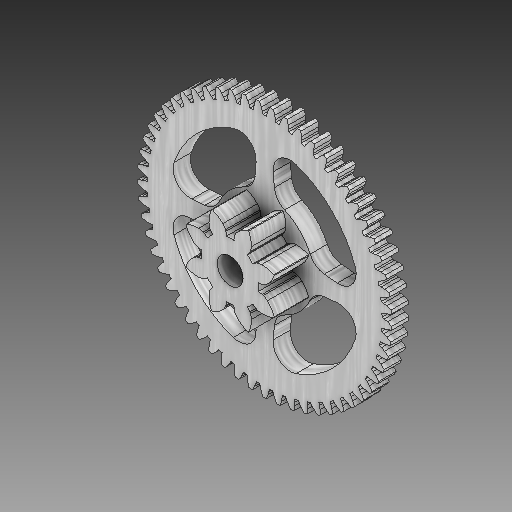
# Autodesk Inventor part: 多段ギアm1.z57,m2.z8
Saved by Autodesk Inventor 2020 (Build 240168000, 168)
## iProperties
Created: 2019-09-05
Part Number: 多段ギアm1.z57,m2.z8
Material: アルミニウム 7075
Document SubType Name: Modeling
Designer: 雪村
Density: 2.81 g/cm^3
Appearance: サテン - ブラシ仕上げ 重厚
Mass: 22.8746 g
Surface Area: 66.3884 cm^2
Volume: 8.14042 cm^3
Description: アルミ7000 12t
Author: 雪村
Autodesk Inventor part; units mm, degrees
(part 1 of 2)
ref_plane "YZ Plane" through (0, 0, 0) normal (1, 0, 0) x (0, 1, 0)
ref_plane "XZ Plane" through (0, 0, 0) normal (0, 1, 0) x (-1, 0, 0)
ref_plane "XY Plane" through (0, 0, 0) normal (0, 0, 1) x (1, 0, 0)
sketch "スケッチ1" plane through (0, 0, 0) normal (0, 0, 1) x (1, 0, 0)
  arc A0 (1.0775, 7.7333) -> (0.985, 7.4527) centre (2.1428, 7.2265) ccw
  arc A1 (1.6924, 8.6387) -> (1.0775, 7.7333) centre (4.1275, 6.3233) ccw
  arc A2 (4.1322, 10.2254) -> (1.6924, 8.6387) centre (6.2553, 4.2918) ccw
  arc A3 (-4.7064, 6.2301) -> (-4.5734, 5.9664) centre (-3.5947, 6.6251) ccw
  arc A4 (-4.9118, 7.3052) -> (-4.7064, 6.2301) centre (-1.5527, 7.3898) ccw
  arc A5 (-4.3085, 10.1524) -> (-4.9118, 7.3052) centre (1.3884, 7.4579) ccw
  arc A6 (-7.7333, 1.0775) -> (-7.4527, 0.985) centre (-7.2265, 2.1428) ccw
  arc A7 (-8.6387, 1.6924) -> (-7.7333, 1.0775) centre (-6.3233, 4.1275) ccw
  arc A8 (-10.2254, 4.1322) -> (-8.6387, 1.6924) centre (-4.2918, 6.2553) ccw
  arc A9 (-6.2301, -4.7064) -> (-5.9664, -4.5734) centre (-6.6251, -3.5947) ccw
  arc A10 (-7.3052, -4.9118) -> (-6.2301, -4.7064) centre (-7.3898, -1.5527) ccw
  arc A11 (-10.1524, -4.3085) -> (-7.3052, -4.9118) centre (-7.4579, 1.3884) ccw
  arc A12 (-1.0775, -7.7333) -> (-0.985, -7.4527) centre (-2.1428, -7.2265) ccw
  arc A13 (-1.6924, -8.6387) -> (-1.0775, -7.7333) centre (-4.1275, -6.3233) ccw
  arc A14 (-4.1322, -10.2254) -> (-1.6924, -8.6387) centre (-6.2553, -4.2918) ccw
  arc A15 (4.7064, -6.2301) -> (4.5734, -5.9664) centre (3.5947, -6.6251) ccw
  arc A16 (4.9118, -7.3052) -> (4.7064, -6.2301) centre (1.5527, -7.3898) ccw
  arc A17 (4.3085, -10.1524) -> (4.9118, -7.3052) centre (-1.3884, -7.4579) ccw
  arc A18 (7.7333, -1.0775) -> (7.4527, -0.985) centre (7.2265, -2.1428) ccw
  arc A19 (8.6387, -1.6924) -> (7.7333, -1.0775) centre (6.3233, -4.1275) ccw
  arc A20 (10.2254, -4.1322) -> (8.6387, -1.6924) centre (4.2918, -6.2553) ccw
  arc A21 (6.2301, 4.7064) -> (5.9664, 4.5734) centre (6.6251, 3.5947) ccw
  arc A22 (7.3052, 4.9118) -> (6.2301, 4.7064) centre (7.3898, 1.5527) ccw
  arc A23 (10.1524, 4.3085) -> (7.3052, 4.9118) centre (7.4579, -1.3884) ccw
  arc A24 (-0.985, 7.4527) -> (-1.0775, 7.7333) centre (-2.1428, 7.2265) ccw
  arc A25 (-1.0775, 7.7333) -> (-1.6924, 8.6387) centre (-4.1275, 6.3233) ccw
  arc A26 (-1.6924, 8.6387) -> (-4.1322, 10.2254) centre (-6.2553, 4.2918) ccw
  arc A27 (-5.9664, 4.5734) -> (-6.2301, 4.7064) centre (-6.6251, 3.5947) ccw
  arc A28 (-6.2301, 4.7064) -> (-7.3052, 4.9118) centre (-7.3898, 1.5527) ccw
  arc A29 (-7.3052, 4.9118) -> (-10.1524, 4.3085) centre (-7.4579, -1.3884) ccw
  arc A30 (-7.4527, -0.985) -> (-7.7333, -1.0775) centre (-7.2265, -2.1428) ccw
  arc A31 (-7.7333, -1.0775) -> (-8.6387, -1.6924) centre (-6.3233, -4.1275) ccw
  arc A32 (-8.6387, -1.6924) -> (-10.2254, -4.1322) centre (-4.2918, -6.2553) ccw
  arc A33 (-4.5734, -5.9664) -> (-4.7064, -6.2301) centre (-3.5947, -6.6251) ccw
  arc A34 (-4.7064, -6.2301) -> (-4.9118, -7.3052) centre (-1.5527, -7.3898) ccw
  arc A35 (-4.9118, -7.3052) -> (-4.3085, -10.1524) centre (1.3884, -7.4579) ccw
  arc A36 (0.985, -7.4527) -> (1.0775, -7.7333) centre (2.1428, -7.2265) ccw
  arc A37 (1.0775, -7.7333) -> (1.6924, -8.6387) centre (4.1275, -6.3233) ccw
  arc A38 (1.6924, -8.6387) -> (4.1322, -10.2254) centre (6.2553, -4.2918) ccw
  arc A39 (5.9664, -4.5734) -> (6.2301, -4.7064) centre (6.6251, -3.5947) ccw
  arc A40 (6.2301, -4.7064) -> (7.3052, -4.9118) centre (7.3898, -1.5527) ccw
  arc A41 (7.3052, -4.9118) -> (10.1524, -4.3085) centre (7.4579, 1.3884) ccw
  arc A42 (7.4527, 0.985) -> (7.7333, 1.0775) centre (7.2265, 2.1428) ccw
  arc A43 (7.7333, 1.0775) -> (8.6387, 1.6924) centre (6.3233, 4.1275) ccw
  arc A44 (8.6387, 1.6924) -> (10.2254, 4.1322) centre (4.2918, 6.2553) ccw
  arc A45 (4.5734, 5.9664) -> (4.7064, 6.2301) centre (3.5947, 6.6251) ccw
  arc A46 (4.7064, 6.2301) -> (4.9118, 7.3052) centre (1.5527, 7.3898) ccw
  arc A47 (4.9118, 7.3052) -> (4.3085, 10.1524) centre (-1.3884, 7.4579) ccw
  arc A48 (0.8647, 6.5431) -> (-0.8647, 6.5431) centre (0, 0) ccw
  arc A49 (-4.0152, 5.2381) -> (-5.2381, 4.0152) centre (0, 0) ccw
  arc A50 (-6.5431, 0.8647) -> (-6.5431, -0.8647) centre (0, 0) ccw
  arc A51 (-5.2381, -4.0152) -> (-4.0152, -5.2381) centre (0, 0) ccw
  arc A52 (-0.8647, -6.5431) -> (0.8647, -6.5431) centre (0, 0) ccw
  arc A53 (4.0152, -5.2381) -> (5.2381, -4.0152) centre (0, 0) ccw
  arc A54 (6.5431, -0.8647) -> (6.5431, 0.8647) centre (0, 0) ccw
  arc A55 (5.2381, 4.0152) -> (4.0152, 5.2381) centre (0, 0) ccw
  arc A56 (-4.1322, 10.2254) -> (-4.3085, 10.1524) centre (0, 0) ccw
  arc A57 (-10.1524, 4.3085) -> (-10.2254, 4.1322) centre (0, 0) ccw
  arc A58 (-10.2254, -4.1322) -> (-10.1524, -4.3085) centre (0, 0) ccw
  arc A59 (-4.3085, -10.1524) -> (-4.1322, -10.2254) centre (0, 0) ccw
  arc A60 (4.1322, -10.2254) -> (4.3085, -10.1524) centre (0, 0) ccw
  arc A61 (10.1524, -4.3085) -> (10.2254, -4.1322) centre (0, 0) ccw
  arc A62 (10.2254, 4.1322) -> (10.1524, 4.3085) centre (0, 0) ccw
  arc A63 (4.3085, 10.1524) -> (4.1322, 10.2254) centre (0, 0) ccw
  line L0 (0.8647, 6.5431) -> (0.985, 7.4527)
  line L1 (-4.0152, 5.2381) -> (-4.5734, 5.9664)
  line L2 (-6.5431, 0.8647) -> (-7.4527, 0.985)
  line L3 (-5.2381, -4.0152) -> (-5.9664, -4.5734)
  line L4 (-0.8647, -6.5431) -> (-0.985, -7.4527)
  line L5 (4.0152, -5.2381) -> (4.5734, -5.9664)
  line L6 (6.5431, -0.8647) -> (7.4527, -0.985)
  line L7 (5.2381, 4.0152) -> (5.9664, 4.5734)
  line L8 (-0.8647, 6.5431) -> (-0.985, 7.4527)
  line L9 (-5.2381, 4.0152) -> (-5.9664, 4.5734)
  line L10 (-6.5431, -0.8647) -> (-7.4527, -0.985)
  line L11 (-4.0152, -5.2381) -> (-4.5734, -5.9664)
  line L12 (0.8647, -6.5431) -> (0.985, -7.4527)
  line L13 (5.2381, -4.0152) -> (5.9664, -4.5734)
  line L14 (6.5431, 0.8647) -> (7.4527, 0.985)
  line L15 (4.0152, 5.2381) -> (4.5734, 5.9664)
  line L16 (-13.0288, 0) -> (13.0288, 0)
  line L17 (0, -13.0288) -> (0, 13.0288)
  line L18 (31.0288, 11.0288) -> (101.0288, 11.0288)
  line L19 (31.0288, 3.0288) -> (101.0288, 3.0288)
  line L20 (31.0288, -4.9712) -> (101.0288, -4.9712)
  line L21 (31.0288, -12.9712) -> (101.0288, -12.9712)
  line L22 (31.0288, -20.9712) -> (101.0288, -20.9712)
  line L23 (31.0288, -28.9712) -> (101.0288, -28.9712)
  line L24 (31.0288, -36.9712) -> (101.0288, -36.9712)
  line L25 (31.0288, -44.9712) -> (101.0288, -44.9712)
  line L26 (31.0288, -52.9712) -> (101.0288, -52.9712)
  line L27 (31.0288, -60.9712) -> (101.0288, -60.9712)
  line L28 (31.0288, -68.9712) -> (101.0288, -68.9712)
  line L29 (31.0288, -76.9712) -> (101.0288, -76.9712)
  line L30 (31.0288, -84.9712) -> (101.0288, -84.9712)
  line L31 (31.0288, 11.0288) -> (31.0288, -84.9712)
  line L32 (101.0288, 11.0288) -> (101.0288, -84.9712)
  line L33 (66.0288, 3.0288) -> (66.0288, -84.9712)
  point P0 (0, 0)
  point P1 (37.0288, 5.0288)
  point P2 (39.5288, -2.9712)
  point P3 (39.5288, -10.9712)
  point P4 (37.0288, -18.9712)
  point P5 (39.5288, -26.9712)
  point P6 (34.5288, -34.9712)
  point P7 (37.0288, -42.9712)
  point P8 (37.0288, -50.9712)
  point P9 (37.0288, -58.9712)
  point P10 (39.5288, -66.9712)
  point P11 (39.5288, -74.9712)
  point P12 (37.0288, -82.9712)
  point P13 (67.0288, -2.9712)
  point P14 (83.2788, -10.9712)
  point P15 (83.2788, -18.9712)
  point P16 (79.5288, -26.9712)
  point P17 (82.0288, -34.9712)
  point P18 (75.7788, -42.9712)
  point P19 (75.7788, -50.9712)
  point P20 (79.5288, -58.9712)
  point P21 (77.0288, -66.9712)
  point P22 (1, 26.5288)
  point P23 (1, 20.5288)
  point P24 (18.25, 26.5288)
  point P25 (20.375, 20.5288)
  constraints: 128 point on circle, 64 centre point, 64 end point, 14 horizontal, 2 midpoint, 2 vertical, 320 other
extrude "押し出し1" add sketch "スケッチ1" along normal blind 8 contours A1 A2 A63 A47 A46 A45 L15 A55 L7 A21 A22 A23 A62 A44 A43 A42 L14 A54 L16 L17 A48 L0 A0 | L17 L16 A50 L2 A6 A7 A8 A57 A29 A28 A27 L9 A49 L1 A3 A4 A5 A56 A26 A25 A24 L8 A48 | L17 A52 L4 A12 A13 A14 A59 A35 A34 A33 L11 A51 L3 A9 A10 A11 A58 A32 A31 A30 L10 A50 L16 | L16 A54 L6 A18 A19 A20 A61 A41 A40 A39 L13 A53 L5 A15 A16 A17 A60 A38 A37 A36 L12 A52 L17
sketch "スケッチ2" plane through (0, 0, 0) normal (0, 0, -1) x (-1, 0, 0)
  arc A0 (0.535, 27.768) -> (0.4038, 27.247) centre (6.485, 25.9929) ccw
  arc A1 (0.7907, 28.5027) -> (0.535, 27.768) centre (8.7588, 25.3182) ccw
  arc A2 (1.2341, 29.4742) -> (0.7907, 28.5027) centre (11.0839, 24.3913) ccw
  arc A3 (-2.523, 27.6583) -> (-2.596, 27.1261) centre (3.5862, 26.5485) ccw
  arc A4 (-2.3497, 28.4167) -> (-2.523, 27.6583) centre (5.9205, 26.128) ccw
  arc A5 (-2.0158, 29.431) -> (-2.3497, 28.4167) centre (8.3334, 25.4626) ccw
  arc A6 (-5.5503, 27.2129) -> (-5.5644, 26.6758) centre (0.6439, 26.7819) ccw
  arc A7 (-5.4615, 27.9857) -> (-5.5503, 27.2129) centre (3.0102, 26.6208) ccw
  arc A8 (-5.2412, 29.0307) -> (-5.4615, 27.9857) centre (5.4817, 26.2248) ccw
  arc A9 (-8.5102, 26.4372) -> (-8.4651, 25.9018) centre (-2.3063, 26.6901) ccw
  arc A10 (-8.507, 27.2151) -> (-8.5102, 26.4372) centre (0.0635, 26.7903) ccw
  arc A11 (-8.403, 28.2779) -> (-8.507, 27.2151) centre (2.5635, 26.6687) ccw
  arc A12 (-11.3669, 25.3405) -> (-11.2632, 24.8134) centre (-5.2284, 26.2744) ccw
  arc A13 (-11.4492, 26.1141) -> (-11.3669, 25.3405) centre (-2.8841, 26.6347) ccw
  arc A14 (-11.4628, 27.1819) -> (-11.4492, 26.1141) centre (-0.3858, 26.7888) ccw
  arc A15 (-14.0856, 23.9363) -> (-13.9245, 23.4237) centre (-8.0871, 25.5398) ccw
  arc A16 (-14.2525, 24.6961) -> (-14.0856, 23.9363) centre (-5.7966, 26.1558) ccw
  arc A17 (-14.3835, 25.7559) -> (-14.2525, 24.6961) centre (-3.3305, 26.5838) ccw
  arc A18 (-16.6333, 22.2415) -> (-16.4168, 21.7498) centre (-10.8476, 24.4952) ccw
  arc A19 (-16.8828, 22.9783) -> (-16.6333, 22.2415) centre (-8.6388, 25.3594) ccw
  arc A20 (-17.1295, 24.0173) -> (-16.8828, 22.9783) centre (-6.2347, 26.0561) ccw
  arc A21 (-18.9791, 20.2767) -> (-18.7098, 19.8118) centre (-13.4764, 23.1532) ccw
  arc A22 (-19.3081, 20.9816) -> (-18.9791, 20.2767) centre (-11.3761, 24.2551) ccw
  arc A23 (-19.6677, 21.9871) -> (-19.3081, 20.9816) centre (-9.0632, 25.2121) ccw
  arc A24 (-21.0945, 18.0658) -> (-20.7757, 17.6333) centre (-15.9417, 21.5301) ccw
  arc A25 (-21.4991, 18.7302) -> (-21.0945, 18.0658) centre (-13.9753, 22.8564) ccw
  arc A26 (-21.9671, 19.69) -> (-21.4991, 18.7302) centre (-11.7818, 24.062) ccw
  arc A27 (-22.9538, 15.6355) -> (-22.5894, 15.2408) centre (-18.2134, 19.6457) ccw
  arc A28 (-23.4291, 16.2514) -> (-22.9538, 15.6355) centre (-16.4049, 21.1803) ccw
  arc A29 (-23.9998, 17.154) -> (-23.4291, 16.2514) centre (-14.3573, 22.6199) ccw
  arc A30 (-24.5345, 13.0155) -> (-24.1289, 12.6632) centre (-20.2641, 17.5229) ccw
  arc A31 (-25.0747, 13.5754) -> (-24.5345, 13.0155) centre (-18.6353, 19.2471) ccw
  arc A32 (-25.7412, 14.4097) -> (-25.0747, 13.5754) centre (-16.7585, 20.9032) ccw
  arc A33 (-25.8175, 10.2375) -> (-25.3755, 9.932) centre (-22.0687, 15.1873) ccw
  arc A34 (-26.4159, 10.7346) -> (-25.8175, 10.2375) centre (-20.6396, 17.0802) ccw
  arc A35 (-27.1702, 11.4905) -> (-26.4159, 10.7346) centre (-18.9563, 18.9327) ccw
  arc A36 (-26.787, 7.3353) -> (-26.3141, 7.0802) centre (-23.6055, 12.6674) ccw
  arc A37 (-27.4364, 7.7635) -> (-26.787, 7.3353) centre (-22.3933, 14.7061) ccw
  arc A38 (-28.2693, 8.4318) -> (-27.4364, 7.7635) centre (-20.924, 16.7325) ccw
  arc A39 (-27.4313, 4.344) -> (-26.9333, 4.1425) centre (-24.8558, 9.9937) ccw
  arc A40 (-28.124, 4.6981) -> (-27.4313, 4.344) centre (-23.8751, 12.1534) ccw
  arc A41 (-29.0253, 5.2708) -> (-28.124, 4.6981) centre (-22.6377, 14.3291) ccw
  arc A42 (-27.7427, 1.2999) -> (-27.2255, 1.1544) centre (-25.8043, 7.1987) ccw
  arc A43 (-28.4701, 1.5757) -> (-27.7427, 1.2999) centre (-25.0672, 9.4531) ccw
  arc A44 (-29.429, 2.0458) -> (-28.4701, 1.5757) centre (-24.0767, 11.7518) ccw
  arc A45 (-27.7173, -1.7599) -> (-27.1873, -1.8476) centre (-26.4396, 4.3163) ccw
  arc A46 (-28.4707, -1.5658) -> (-27.7173, -1.7599) centre (-25.955, 6.6382) ccw
  arc A47 (-29.4754, -1.2041) -> (-28.4707, -1.5658) centre (-25.2233, 9.0318) ccw
  arc A48 (-27.3555, -4.7983) -> (-26.819, -4.8272) centre (-26.754, 1.3816) ccw
  arc A49 (-28.1256, -4.6883) -> (-27.3555, -4.7983) centre (-26.5277, 3.7426) ccw
  arc A50 (-29.1641, -4.4393) -> (-28.1256, -4.6883) centre (-26.0638, 6.2023) ccw
  arc A51 (-26.6616, -7.7786) -> (-26.1252, -7.7482) centre (-26.7436, -1.57) ccw
  arc A52 (-27.4392, -7.7539) -> (-26.6616, -7.7786) centre (-26.7784, 0.8016) ccw
  arc A53 (-28.4987, -7.6207) -> (-27.4392, -7.7539) centre (-26.5879, 3.2974) ccw
  arc A54 (-25.6441, -10.6643) -> (-25.1143, -10.5752) centre (-26.4085, -4.5025) ccw
  arc A55 (-26.4196, -10.7253) -> (-25.6441, -10.6643) centre (-26.7041, -2.1491) ccw
  arc A56 (-27.4874, -10.7095) -> (-26.4196, -10.7253) centre (-26.7893, 0.3525) ccw
  arc A57 (-24.3153, -13.4207) -> (-23.7985, -13.2738) centre (-25.7529, -7.3803) ccw
  arc A58 (-25.0794, -13.5666) -> (-24.3153, -13.4207) centre (-26.3056, -5.0737) ccw
  arc A59 (-26.1424, -13.6683) -> (-25.0794, -13.5666) centre (-26.6655, -2.5967) ccw
  arc A60 (-22.6913, -16.0141) -> (-22.1938, -15.8113) centre (-24.7848, -10.1685) ccw
  arc A61 (-23.4347, -16.2432) -> (-22.6913, -16.0141) centre (-25.5878, -7.9368) ccw
  arc A62 (-24.4801, -16.4613) -> (-23.4347, -16.2432) centre (-26.218, -5.5144) ccw
  arc A63 (-20.7919, -18.4131) -> (-20.3198, -18.1568) centre (-23.5157, -12.8333) ccw
  arc A64 (-21.5056, -18.7227) -> (-20.7919, -18.4131) centre (-24.5594, -10.7034) ccw
  arc A65 (-22.5207, -19.0544) -> (-21.5056, -18.7227) centre (-25.4522, -8.3651) ccw
  arc A66 (-18.6401, -20.5887) -> (-18.1991, -20.2819) centre (-21.9612, -15.3424) ccw
  arc A67 (-19.3155, -20.9748) -> (-18.6401, -20.5887) centre (-23.2328, -13.3402) ccw
  arc A68 (-20.2879, -21.4162) -> (-19.3155, -20.9748) centre (-24.3775, -11.1143) ccw
  arc A69 (-16.2621, -22.5143) -> (-15.8574, -22.1609) centre (-20.1401, -17.6652) ccw
  arc A70 (-16.8908, -22.9724) -> (-16.2621, -22.5143) centre (-21.6243, -15.8151) ccw
  arc A71 (-17.8088, -23.518) -> (-16.8908, -22.9724) centre (-23.0069, -13.7285) ccw
  arc A72 (-13.6866, -24.1666) -> (-13.3233, -23.7708) centre (-18.0746, -19.7735) ccw
  arc A73 (-14.2612, -24.6911) -> (-13.6866, -24.1666) centre (-19.7533, -18.0979) ccw
  arc A74 (-15.1135, -25.3344) -> (-14.2612, -24.6911) centre (-21.357, -16.1762) ccw
  arc A75 (-10.945, -25.5256) -> (-10.6274, -25.0922) centre (-15.7896, -21.6419) ccw
  arc A76 (-11.4584, -26.1101) -> (-10.945, -25.5256) centre (-17.6425, -20.1611) ccw
  arc A77 (-12.2348, -26.8433) -> (-11.4584, -26.1101) centre (-19.4479, -18.4274) ccw
  arc A78 (-8.0706, -26.5747) -> (-7.8026, -26.109) centre (-13.313, -23.2475) ccw
  arc A79 (-8.5165, -27.2121) -> (-8.0706, -26.5747) centre (-15.3175, -21.9796) ccw
  arc A80 (-9.2075, -28.0263) -> (-8.5165, -27.2121) centre (-17.3027, -20.455) ccw
  arc A81 (-5.0982, -27.3012) -> (-4.883, -26.8089) centre (-10.6748, -24.571) ccw
  arc A82 (-5.4713, -27.9838) -> (-5.0982, -27.3012) centre (-12.8066, -23.5312) ccw
  arc A83 (-6.0685, -28.8691) -> (-5.4713, -27.9838) centre (-14.9474, -22.2343) ccw
  arc A84 (-2.0639, -27.6964) -> (-1.9042, -27.1834) centre (-7.907, -25.5961) ccw
  arc A85 (-2.3596, -28.4159) -> (-2.0639, -27.6964) centre (-10.1402, -24.7972) ccw
  arc A86 (-2.8559, -29.3614) -> (-2.3596, -28.4159) centre (-12.4108, -23.7437) ccw
  arc A87 (0.9955, -27.7553) -> (1.0978, -27.2279) centre (-5.0432, -26.3106) ccw
  arc A88 (0.7807, -28.503) -> (0.9955, -27.7553) centre (-7.3508, -25.7622) ccw
  arc A89 (0.3915, -29.4974) -> (0.7807, -28.503) centre (-9.7234, -24.9649) ccw
  arc A90 (4.0428, -27.4773) -> (4.0864, -26.9419) centre (-2.1182, -26.7057) ccw
  arc A91 (3.9115, -28.2441) -> (4.0428, -27.4773) centre (-4.4721, -26.4145) ccw
  arc A92 (3.634, -29.2753) -> (3.9115, -28.2441) centre (-6.9181, -25.883) ccw
  arc A93 (7.041, -26.8658) -> (7.0254, -26.3288) centre (0.8325, -26.7767) ccw
  arc A94 (6.9957, -27.6348) -> (7.041, -26.8658) centre (-1.5392, -26.7462) ccw
  arc A95 (6.8325, -28.6979) -> (6.9957, -27.6348) centre (-4.0287, -26.487) ccw
  arc A96 (9.9537, -25.9282) -> (9.8792, -25.3962) centre (3.7731, -26.5226) ccw
  arc A97 (9.9933, -26.7051) -> (9.9537, -25.9282) centre (1.4125, -26.7532) ccw
  arc A98 (9.948, -27.772) -> (9.9933, -26.7051) centre (-1.0905, -26.7694) ccw
  arc A99 (12.7456, -24.6759) -> (12.613, -24.1552) centre (6.6679, -25.9465) ccw
  arc A100 (12.8704, -25.4437) -> (12.7456, -24.6759) centre (4.347, -26.4354) ccw
  arc A101 (12.9428, -26.5091) -> (12.8704, -25.4437) centre (1.861, -26.7269) ccw
  arc A102 (15.3828, -23.124) -> (15.1937, -22.6211) centre (9.4817, -25.0555) ccw
  arc A103 (15.5913, -23.8734) -> (15.3828, -23.124) centre (7.2287, -25.7968) ccw
  arc A104 (15.7805, -24.9244) -> (15.5913, -23.8734) centre (4.7899, -26.36) ccw
  arc A105 (17.8332, -21.2914) -> (17.59, -20.8124) centre (12.1805, -23.8604) ccw
  arc A106 (18.123, -22.0133) -> (17.8332, -21.2914) centre (10.0227, -24.845) ccw
  arc A107 (18.4266, -23.0372) -> (18.123, -22.0133) centre (7.6606, -25.6731) ccw
  arc A108 (20.0672, -19.2004) -> (19.7728, -18.751) centre (14.7314, -22.3756) ccw
  arc A109 (20.4346, -19.8861) -> (20.0672, -19.2004) centre (12.695, -23.5916) ccw
  arc A110 (20.849, -20.8703) -> (20.4346, -19.8861) centre (10.4383, -24.6745) ccw
  arc A111 (22.0576, -16.8763) -> (21.7155, -16.462) centre (17.1035, -20.6192) ccw
  arc A112 (22.4982, -17.5174) -> (22.0576, -16.8763) centre (15.2132, -22.0519) ccw
  arc A113 (23.0184, -18.45) -> (22.4982, -17.5174) centre (13.0894, -23.3764) ccw
  arc A114 (23.7803, -14.3473) -> (23.3947, -13.9732) centre (19.268, -18.6126) ccw
  arc A115 (24.2887, -14.9361) -> (23.7803, -14.3473) centre (17.5468, -20.2445) ccw
  arc A116 (24.9083, -15.8058) -> (24.2887, -14.9361) centre (15.5815, -21.7946) ccw
  arc A117 (25.2143, -11.6442) -> (24.7899, -11.3148) centre (21.1986, -16.38) ccw
  arc A118 (25.7844, -12.1735) -> (25.2143, -11.6442) centre (19.6673, -18.1913) ccw
  arc A119 (26.4959, -12.9698) -> (25.7844, -12.1735) centre (17.8846, -19.9482) ccw
  arc A120 (26.3422, -8.7998) -> (25.8841, -8.519) centre (22.8719, -13.9485) ccw
  arc A121 (26.9671, -9.2631) -> (26.3422, -8.7998) centre (21.5491, -15.9173) ccw
  arc A122 (27.7619, -9.9763) -> (26.9671, -9.2631) centre (19.9705, -17.8597) ccw
  arc A123 (27.1504, -5.8485) -> (26.6642, -5.6199) centre (24.2675, -11.3478) ccw
  arc A124 (27.8224, -6.2403) -> (27.1504, -5.8485) centre (23.1694, -13.4501) ccw
  arc A125 (28.6909, -6.8617) -> (27.8224, -6.2403) centre (21.814, -15.5544) ccw
  arc A126 (27.629, -2.8262) -> (27.1206, -2.6525) centre (25.3685, -8.6093) ccw
  arc A127 (28.3401, -3.1417) -> (27.629, -2.8262) centre (24.5084, -10.8197) ccw
  arc A128 (29.2716, -3.6638) -> (28.3401, -3.1417) centre (23.3927, -13.0603) ccw
  arc A129 (27.7722, 0.2303) -> (27.2478, 0.3471) centre (26.1617, -5.7663) ccw
  arc A130 (28.5137, -0.005) -> (27.7722, 0.2303) centre (25.5499, -8.0579) ccw
  arc A131 (29.497, -0.4215) -> (28.5137, -0.005) centre (24.6875, -10.4076) ccw
  arc A132 (27.5783, 3.2841) -> (27.0442, 3.3425) centre (26.6372, -2.8533) ccw
  arc A133 (28.3412, 3.1318) -> (27.5783, 3.2841) centre (26.2813, -5.1983) ccw
  arc A134 (29.3643, 2.826) -> (28.3412, 3.1318) centre (25.6826, -7.6286) ccw
  arc A135 (27.0496, 6.298) -> (26.5124, 6.2973) centre (26.7894, 0.0943) ccw
  arc A136 (27.8246, 6.2305) -> (27.0496, 6.298) centre (26.6936, -2.2756) ccw
  arc A137 (28.8752, 6.0392) -> (27.8246, 6.2305) centre (26.3659, -4.757) ccw
  arc A138 (26.1926, 9.2355) -> (25.6587, 9.1756) centre (26.6165, 3.0408) ccw
  arc A139 (26.9703, 9.2537) -> (26.1926, 9.2355) centre (26.7819, 0.6748) ccw
  arc A140 (28.0356, 9.179) -> (26.9703, 9.2537) centre (26.7292, -1.8277) ccw
  arc A141 (25.0177, 12.0608) -> (24.4936, 11.9426) centre (26.1204, 5.9504) ccw
  arc A142 (25.7887, 12.1645) -> (25.0177, 12.0608) centre (26.5451, 3.6169) ccw
  arc A143 (26.8557, 12.2075) -> (25.7887, 12.1645) centre (26.768, 1.1238) ccw
  arc A144 (23.5391, 14.7398) -> (23.0312, 14.5646) centre (25.3073, 8.7878) ccw
  arc A145 (24.294, 14.9276) -> (23.5391, 14.7398) centre (25.9861, 6.5151) ccw
  arc A146 (25.3498, 15.0877) -> (24.294, 14.9276) centre (26.4819, 4.0617) ccw
  arc A147 (21.7747, 17.2398) -> (21.2891, 17.0099) centre (24.187, 11.5184) ccw
  arc A148 (22.4971, 17.5072) -> (21.7747, 17.2398) centre (25.1117, 9.3343) ccw
  arc A149 (23.5361, 17.7848) -> (22.4971, 17.5072) centre (25.8744, 6.9503) ccw
  arc A150 (19.746, 19.5306) -> (19.2887, 19.2486) centre (22.773, 14.1093) ccw
  arc A151 (20.4346, 19.8758) -> (19.746, 19.5306) centre (23.9325, 12.0401) ccw
  arc A152 (21.4368, 20.2661) -> (20.4346, 19.8758) centre (24.9528, 9.7545) ccw
  arc A153 (17.4777, 21.5843) -> (17.0541, 21.2537) centre (21.0827, 16.5289) ccw
  arc A154 (18.1241, 22.0031) -> (17.4777, 21.5843) centre (22.4627, 14.5998) ccw
  arc A155 (19.0773, 22.5013) -> (18.1241, 22.0031) centre (23.7282, 12.4403) ccw
  arc A156 (14.9971, 23.3759) -> (14.6125, 23.0008) centre (19.1364, 18.7478) ccw
  arc A157 (15.5935, 23.8634) -> (14.9971, 23.3759) centre (20.7203, 16.9823) ccw
  arc A158 (16.4862, 24.4634) -> (15.5935, 23.8634) centre (22.2157, 14.9751) ccw
  arc A159 (12.3346, 24.8839) -> (11.9936, 24.4687) centre (16.9579, 20.7392) ccw
  arc A160 (12.8793, 25.4392) -> (12.3346, 24.8839) centre (18.7263, 19.1586) ccw
  arc A161 (13.6949, 26.1285) -> (12.8793, 25.4392) centre (20.4335, 17.3281) ccw
  arc A162 (9.5223, 26.0897) -> (9.229, 25.6396) centre (14.5734, 22.4788) ccw
  arc A163 (10.0026, 26.7016) -> (9.5223, 26.0897) centre (16.505, 21.1024) ccw
  arc A164 (10.7375, 27.4765) -> (10.0026, 26.7016) centre (18.4032, 19.4708) ccw
  arc A165 (6.5944, 26.9789) -> (6.3525, 26.4992) centre (12.0121, 23.9456) ccw
  arc A166 (7.0045, 27.6399) -> (6.5944, 26.9789) centre (14.0834, 22.79) ccw
  arc A167 (7.6497, 28.4909) -> (7.0045, 27.6399) centre (16.1496, 21.3771) ccw
  arc A168 (3.5865, 27.5406) -> (3.3988, 27.0372) centre (9.305, 25.1217) ccw
  arc A169 (3.9214, 28.2427) -> (3.5865, 27.5406) centre (11.4909, 24.201) ccw
  arc A170 (4.469, 29.1595) -> (3.9214, 28.2427) centre (13.6999, 23.024) ccw
  arc A171 (-0.4038, 27.247) -> (-0.535, 27.768) centre (-6.485, 25.9929) ccw
  arc A172 (-0.535, 27.768) -> (-0.7907, 28.5027) centre (-8.7588, 25.3182) ccw
  arc A173 (-0.7907, 28.5027) -> (-1.2341, 29.4742) centre (-11.0839, 24.3913) ccw
  arc A174 (-3.3988, 27.0372) -> (-3.5865, 27.5406) centre (-9.305, 25.1217) ccw
  arc A175 (-3.5865, 27.5406) -> (-3.9214, 28.2427) centre (-11.4909, 24.201) ccw
  arc A176 (-3.9214, 28.2427) -> (-4.469, 29.1595) centre (-13.6999, 23.024) ccw
  arc A177 (-6.3525, 26.4992) -> (-6.5944, 26.9789) centre (-12.0121, 23.9456) ccw
  arc A178 (-6.5944, 26.9789) -> (-7.0045, 27.6399) centre (-14.0834, 22.79) ccw
  arc A179 (-7.0045, 27.6399) -> (-7.6497, 28.4909) centre (-16.1496, 21.3771) ccw
  arc A180 (-9.229, 25.6396) -> (-9.5223, 26.0897) centre (-14.5734, 22.4788) ccw
  arc A181 (-9.5223, 26.0897) -> (-10.0026, 26.7016) centre (-16.505, 21.1024) ccw
  arc A182 (-10.0026, 26.7016) -> (-10.7375, 27.4765) centre (-18.4032, 19.4708) ccw
  arc A183 (-11.9936, 24.4687) -> (-12.3346, 24.8839) centre (-16.9579, 20.7392) ccw
  arc A184 (-12.3346, 24.8839) -> (-12.8793, 25.4392) centre (-18.7263, 19.1586) ccw
  arc A185 (-12.8793, 25.4392) -> (-13.6949, 26.1285) centre (-20.4335, 17.3281) ccw
  arc A186 (-14.6125, 23.0008) -> (-14.9971, 23.3759) centre (-19.1364, 18.7478) ccw
  arc A187 (-14.9971, 23.3759) -> (-15.5997, 23.868) centre (-20.7203, 16.9823) ccw
  arc A188 (-15.5997, 23.868) -> (-16.4862, 24.4634) centre (-22.2157, 14.9751) ccw
  arc A189 (-17.0541, 21.2537) -> (-17.4777, 21.5843) centre (-21.0827, 16.5289) ccw
  arc A190 (-17.4777, 21.5843) -> (-18.1307, 22.007) centre (-22.4627, 14.5998) ccw
  arc A191 (-18.1307, 22.007) -> (-19.0773, 22.5013) centre (-23.7282, 12.4403) ccw
  arc A192 (-19.2887, 19.2486) -> (-19.746, 19.5306) centre (-22.773, 14.1093) ccw
  arc A193 (-19.746, 19.5306) -> (-20.4416, 19.8789) centre (-23.9325, 12.0401) ccw
  arc A194 (-20.4416, 19.8789) -> (-21.4368, 20.2661) centre (-24.9528, 9.7545) ccw
  arc A195 (-21.2891, 17.0099) -> (-21.7747, 17.2398) centre (-24.187, 11.5184) ccw
  arc A196 (-21.7747, 17.2398) -> (-22.5044, 17.5095) centre (-25.1117, 9.3343) ccw
  arc A197 (-22.5044, 17.5095) -> (-23.5361, 17.7848) centre (-25.8744, 6.9503) ccw
  arc A198 (-23.0312, 14.5646) -> (-23.5391, 14.7398) centre (-25.3073, 8.7878) ccw
  arc A199 (-23.5391, 14.7398) -> (-24.294, 14.9276) centre (-25.9861, 6.5151) ccw
  arc A200 (-24.294, 14.9276) -> (-25.3498, 15.0877) centre (-26.4819, 4.0617) ccw
  arc A201 (-24.4936, 11.9426) -> (-25.0177, 12.0608) centre (-26.1204, 5.9504) ccw
  arc A202 (-25.0177, 12.0608) -> (-25.7887, 12.1645) centre (-26.5451, 3.6169) ccw
  arc A203 (-25.7887, 12.1645) -> (-26.8557, 12.2075) centre (-26.768, 1.1238) ccw
  arc A204 (-25.6587, 9.1756) -> (-26.1926, 9.2355) centre (-26.6165, 3.0408) ccw
  arc A205 (-26.1926, 9.2355) -> (-26.9703, 9.2537) centre (-26.7819, 0.6748) ccw
  arc A206 (-26.9703, 9.2537) -> (-28.0356, 9.179) centre (-26.7292, -1.8277) ccw
  arc A207 (-26.5124, 6.2973) -> (-27.0496, 6.298) centre (-26.7894, 0.0943) ccw
  arc A208 (-27.0496, 6.298) -> (-27.8246, 6.2305) centre (-26.6936, -2.2756) ccw
  arc A209 (-27.8246, 6.2305) -> (-28.8752, 6.0392) centre (-26.3659, -4.757) ccw
  arc A210 (-27.0442, 3.3425) -> (-27.5783, 3.2841) centre (-26.6372, -2.8533) ccw
  arc A211 (-27.5783, 3.2841) -> (-28.3412, 3.1318) centre (-26.2813, -5.1983) ccw
  arc A212 (-28.3412, 3.1318) -> (-29.3643, 2.826) centre (-25.6826, -7.6286) ccw
  arc A213 (-27.2478, 0.3471) -> (-27.7722, 0.2303) centre (-26.1617, -5.7663) ccw
  arc A214 (-27.7722, 0.2303) -> (-28.5065, -0.0023) centre (-25.5499, -8.0579) ccw
  arc A215 (-28.5065, -0.0023) -> (-29.497, -0.4215) centre (-24.6875, -10.4076) ccw
  arc A216 (-27.1206, -2.6525) -> (-27.629, -2.8262) centre (-25.3685, -8.6093) ccw
  arc A217 (-27.629, -2.8262) -> (-28.3332, -3.1383) centre (-24.5084, -10.8197) ccw
  arc A218 (-28.3332, -3.1383) -> (-29.2716, -3.6638) centre (-23.3927, -13.0603) ccw
  arc A219 (-26.6642, -5.6199) -> (-27.1504, -5.8485) centre (-24.2675, -11.3478) ccw
  arc A220 (-27.1504, -5.8485) -> (-27.8224, -6.2403) centre (-23.1694, -13.4501) ccw
  arc A221 (-27.8224, -6.2403) -> (-28.6909, -6.8617) centre (-21.814, -15.5544) ccw
  arc A222 (-25.8841, -8.519) -> (-26.3422, -8.7998) centre (-22.8719, -13.9485) ccw
  arc A223 (-26.3422, -8.7998) -> (-26.9671, -9.2631) centre (-21.5491, -15.9173) ccw
  arc A224 (-26.9671, -9.2631) -> (-27.7619, -9.9763) centre (-19.9705, -17.8597) ccw
  arc A225 (-24.7899, -11.3148) -> (-25.2143, -11.6442) centre (-21.1986, -16.38) ccw
  arc A226 (-25.2143, -11.6442) -> (-25.7844, -12.1735) centre (-19.6673, -18.1913) ccw
  arc A227 (-25.7844, -12.1735) -> (-26.4959, -12.9698) centre (-17.8846, -19.9482) ccw
  arc A228 (-23.3947, -13.9732) -> (-23.7803, -14.3473) centre (-19.268, -18.6126) ccw
  arc A229 (-23.7803, -14.3473) -> (-24.2887, -14.9361) centre (-17.5468, -20.2445) ccw
  arc A230 (-24.2887, -14.9361) -> (-24.9083, -15.8058) centre (-15.5815, -21.7946) ccw
  arc A231 (-21.7155, -16.462) -> (-22.0576, -16.8763) centre (-17.1035, -20.6192) ccw
  arc A232 (-22.0576, -16.8763) -> (-22.4982, -17.5174) centre (-15.2132, -22.0519) ccw
  arc A233 (-22.4982, -17.5174) -> (-23.0184, -18.45) centre (-13.0894, -23.3764) ccw
  arc A234 (-19.7728, -18.751) -> (-20.0672, -19.2004) centre (-14.7314, -22.3756) ccw
  arc A235 (-20.0672, -19.2004) -> (-20.4313, -19.8792) centre (-12.695, -23.5916) ccw
  arc A236 (-20.4313, -19.8792) -> (-20.849, -20.8703) centre (-10.4383, -24.6745) ccw
  arc A237 (-17.59, -20.8124) -> (-17.8332, -21.2914) centre (-12.1805, -23.8604) ccw
  arc A238 (-17.8332, -21.2914) -> (-18.123, -22.0134) centre (-10.0227, -24.845) ccw
  arc A239 (-18.123, -22.0134) -> (-18.4266, -23.0372) centre (-7.6606, -25.6731) ccw
  arc A240 (-15.1937, -22.6211) -> (-15.3828, -23.124) centre (-9.4817, -25.0555) ccw
  arc A241 (-15.3828, -23.124) -> (-15.5913, -23.8734) centre (-7.2287, -25.7968) ccw
  arc A242 (-15.5913, -23.8734) -> (-15.7805, -24.9244) centre (-4.7899, -26.36) ccw
  arc A243 (-12.613, -24.1552) -> (-12.7456, -24.6759) centre (-6.6679, -25.9465) ccw
  arc A244 (-12.7456, -24.6759) -> (-12.8704, -25.4437) centre (-4.347, -26.4354) ccw
  arc A245 (-12.8704, -25.4437) -> (-12.9428, -26.5091) centre (-1.861, -26.7269) ccw
  arc A246 (-9.8792, -25.3962) -> (-9.9537, -25.9282) centre (-3.7731, -26.5226) ccw
  arc A247 (-9.9537, -25.9282) -> (-9.9933, -26.7051) centre (-1.4125, -26.7532) ccw
  arc A248 (-9.9933, -26.7051) -> (-9.948, -27.772) centre (1.0905, -26.7694) ccw
  arc A249 (-7.0254, -26.3288) -> (-7.041, -26.8658) centre (-0.8325, -26.7767) ccw
  arc A250 (-7.041, -26.8658) -> (-6.9949, -27.6424) centre (1.5392, -26.7462) ccw
  arc A251 (-6.9949, -27.6424) -> (-6.8325, -28.6979) centre (4.0287, -26.487) ccw
  arc A252 (-4.0864, -26.9419) -> (-4.0428, -27.4773) centre (2.1182, -26.7057) ccw
  arc A253 (-4.0428, -27.4773) -> (-3.9115, -28.2441) centre (4.4721, -26.4145) ccw
  arc A254 (-3.9115, -28.2441) -> (-3.634, -29.2753) centre (6.9181, -25.883) ccw
  arc A255 (-1.0978, -27.2279) -> (-0.9955, -27.7553) centre (5.0432, -26.3106) ccw
  arc A256 (-0.9955, -27.7553) -> (-0.7807, -28.503) centre (7.3508, -25.7622) ccw
  arc A257 (-0.7807, -28.503) -> (-0.3915, -29.4974) centre (9.7234, -24.9649) ccw
  arc A258 (1.9042, -27.1834) -> (2.0639, -27.6964) centre (7.907, -25.5961) ccw
  arc A259 (2.0639, -27.6964) -> (2.3596, -28.4159) centre (10.1402, -24.7972) ccw
  arc A260 (2.3596, -28.4159) -> (2.8559, -29.3614) centre (12.4108, -23.7437) ccw
  arc A261 (4.883, -26.8089) -> (5.0982, -27.3012) centre (10.6748, -24.571) ccw
  arc A262 (5.0982, -27.3012) -> (5.4713, -27.9838) centre (12.8066, -23.5312) ccw
  arc A263 (5.4713, -27.9838) -> (6.0685, -28.8691) centre (14.9474, -22.2343) ccw
  arc A264 (7.8026, -26.109) -> (8.0706, -26.5747) centre (13.313, -23.2475) ccw
  arc A265 (8.0706, -26.5747) -> (8.5165, -27.2121) centre (15.3175, -21.9796) ccw
  arc A266 (8.5165, -27.2121) -> (9.2075, -28.0263) centre (17.3027, -20.455) ccw
  arc A267 (10.6274, -25.0922) -> (10.945, -25.5256) centre (15.7896, -21.6419) ccw
  arc A268 (10.945, -25.5256) -> (11.4584, -26.1101) centre (17.6425, -20.1611) ccw
  arc A269 (11.4584, -26.1101) -> (12.2348, -26.8433) centre (19.4479, -18.4274) ccw
  arc A270 (13.3233, -23.7708) -> (13.6866, -24.1666) centre (18.0746, -19.7735) ccw
  arc A271 (13.6866, -24.1666) -> (14.2612, -24.6911) centre (19.7533, -18.0979) ccw
  arc A272 (14.2612, -24.6911) -> (15.1135, -25.3344) centre (21.357, -16.1762) ccw
  arc A273 (15.8574, -22.1609) -> (16.2621, -22.5143) centre (20.1401, -17.6652) ccw
  arc A274 (16.2621, -22.5143) -> (16.8908, -22.9724) centre (21.6243, -15.8151) ccw
  arc A275 (16.8908, -22.9724) -> (17.8088, -23.518) centre (23.0069, -13.7285) ccw
  arc A276 (18.1991, -20.2819) -> (18.6401, -20.5887) centre (21.9612, -15.3424) ccw
  arc A277 (18.6401, -20.5887) -> (19.3155, -20.9748) centre (23.2328, -13.3402) ccw
  arc A278 (19.3155, -20.9748) -> (20.2879, -21.4162) centre (24.3775, -11.1143) ccw
  arc A279 (20.3198, -18.1568) -> (20.7919, -18.4131) centre (23.5157, -12.8333) ccw
  arc A280 (20.7919, -18.4131) -> (21.5056, -18.7227) centre (24.5594, -10.7034) ccw
  arc A281 (21.5056, -18.7227) -> (22.5207, -19.0544) centre (25.4522, -8.3651) ccw
  arc A282 (22.1938, -15.8113) -> (22.6913, -16.0141) centre (24.7848, -10.1685) ccw
  arc A283 (22.6913, -16.0141) -> (23.4347, -16.2432) centre (25.5878, -7.9368) ccw
  arc A284 (23.4347, -16.2432) -> (24.4801, -16.4613) centre (26.218, -5.5144) ccw
  arc A285 (23.7985, -13.2738) -> (24.3153, -13.4207) centre (25.7529, -7.3803) ccw
  arc A286 (24.3153, -13.4207) -> (25.0794, -13.5666) centre (26.3056, -5.0737) ccw
  arc A287 (25.0794, -13.5666) -> (26.1424, -13.6683) centre (26.6655, -2.5967) ccw
  arc A288 (25.1143, -10.5752) -> (25.6441, -10.6643) centre (26.4085, -4.5025) ccw
  arc A289 (25.6441, -10.6643) -> (26.4196, -10.7253) centre (26.7041, -2.1491) ccw
  arc A290 (26.4196, -10.7253) -> (27.4874, -10.7095) centre (26.7893, 0.3525) ccw
  arc A291 (26.1252, -7.7482) -> (26.6616, -7.7786) centre (26.7436, -1.57) ccw
  arc A292 (26.6616, -7.7786) -> (27.4392, -7.7539) centre (26.7784, 0.8016) ccw
  arc A293 (27.4392, -7.7539) -> (28.4987, -7.6207) centre (26.5879, 3.2974) ccw
  arc A294 (26.819, -4.8272) -> (27.3555, -4.7983) centre (26.754, 1.3816) ccw
  arc A295 (27.3555, -4.7983) -> (28.1256, -4.6883) centre (26.5277, 3.7426) ccw
  arc A296 (28.1256, -4.6883) -> (29.1641, -4.4393) centre (26.0638, 6.2023) ccw
  arc A297 (27.1873, -1.8476) -> (27.7173, -1.7599) centre (26.4396, 4.3163) ccw
  arc A298 (27.7173, -1.7599) -> (28.4706, -1.5658) centre (25.955, 6.6382) ccw
  arc A299 (28.4706, -1.5658) -> (29.4754, -1.2041) centre (25.2233, 9.0318) ccw
  arc A300 (27.2255, 1.1544) -> (27.7427, 1.2999) centre (25.8043, 7.1987) ccw
  arc A301 (27.7427, 1.2999) -> (28.4631, 1.5727) centre (25.0672, 9.4531) ccw
  arc A302 (28.4631, 1.5727) -> (29.429, 2.0458) centre (24.0767, 11.7518) ccw
  arc A303 (26.9333, 4.1425) -> (27.4313, 4.344) centre (24.8558, 9.9937) ccw
  arc A304 (27.4313, 4.344) -> (28.124, 4.6981) centre (23.8751, 12.1534) ccw
  arc A305 (28.124, 4.6981) -> (29.0253, 5.2708) centre (22.6377, 14.3291) ccw
  arc A306 (26.3141, 7.0802) -> (26.787, 7.3353) centre (23.6055, 12.6674) ccw
  arc A307 (26.787, 7.3353) -> (27.4364, 7.7635) centre (22.3933, 14.7061) ccw
  arc A308 (27.4364, 7.7635) -> (28.2693, 8.4318) centre (20.924, 16.7325) ccw
  arc A309 (25.3755, 9.932) -> (25.8175, 10.2375) centre (22.0687, 15.1873) ccw
  arc A310 (25.8175, 10.2375) -> (26.4159, 10.7346) centre (20.6396, 17.0802) ccw
  arc A311 (26.4159, 10.7346) -> (27.1702, 11.4905) centre (18.9563, 18.9327) ccw
  arc A312 (24.1289, 12.6632) -> (24.5345, 13.0155) centre (20.2641, 17.5229) ccw
  arc A313 (24.5345, 13.0155) -> (25.0747, 13.5754) centre (18.6353, 19.2471) ccw
  arc A314 (25.0747, 13.5754) -> (25.7412, 14.4097) centre (16.7585, 20.9032) ccw
  arc A315 (22.5894, 15.2408) -> (22.9538, 15.6355) centre (18.2134, 19.6457) ccw
  arc A316 (22.9538, 15.6355) -> (23.4247, 16.2452) centre (16.4049, 21.1803) ccw
  arc A317 (23.4247, 16.2452) -> (23.9998, 17.154) centre (14.3573, 22.6199) ccw
  arc A318 (20.7757, 17.6333) -> (21.0945, 18.0658) centre (15.9417, 21.5301) ccw
  arc A319 (21.0945, 18.0658) -> (21.4954, 18.7235) centre (13.9753, 22.8564) ccw
  arc A320 (21.4954, 18.7235) -> (21.9671, 19.69) centre (11.7818, 24.062) ccw
  arc A321 (18.7098, 19.8118) -> (18.9791, 20.2767) centre (13.4764, 23.1532) ccw
  arc A322 (18.9791, 20.2767) -> (19.3081, 20.9816) centre (11.3761, 24.2551) ccw
  arc A323 (19.3081, 20.9816) -> (19.6677, 21.9871) centre (9.0632, 25.2121) ccw
  arc A324 (16.4168, 21.7498) -> (16.6333, 22.2415) centre (10.8476, 24.4952) ccw
  arc A325 (16.6333, 22.2415) -> (16.8828, 22.9783) centre (8.6388, 25.3594) ccw
  arc A326 (16.8828, 22.9783) -> (17.1295, 24.0173) centre (6.2347, 26.0561) ccw
  arc A327 (13.9245, 23.4237) -> (14.0856, 23.9363) centre (8.0871, 25.5398) ccw
  arc A328 (14.0856, 23.9363) -> (14.2525, 24.6961) centre (5.7966, 26.1558) ccw
  arc A329 (14.2525, 24.6961) -> (14.3835, 25.7559) centre (3.3305, 26.5838) ccw
  arc A330 (11.2632, 24.8134) -> (11.3669, 25.3405) centre (5.2284, 26.2744) ccw
  arc A331 (11.3669, 25.3405) -> (11.4492, 26.1141) centre (2.8841, 26.6347) ccw
  arc A332 (11.4492, 26.1141) -> (11.4628, 27.1819) centre (0.3858, 26.7888) ccw
  arc A333 (8.4651, 25.9018) -> (8.5102, 26.4372) centre (2.3063, 26.6901) ccw
  arc A334 (8.5102, 26.4372) -> (8.507, 27.2151) centre (-0.0635, 26.7903) ccw
  arc A335 (8.507, 27.2151) -> (8.403, 28.2779) centre (-2.5635, 26.6687) ccw
  arc A336 (5.5644, 26.6758) -> (5.5503, 27.2129) centre (-0.6439, 26.7819) ccw
  arc A337 (5.5503, 27.2129) -> (5.4615, 27.9857) centre (-3.0102, 26.6208) ccw
  arc A338 (5.4615, 27.9857) -> (5.2412, 29.0307) centre (-5.4817, 26.2248) ccw
  arc A339 (2.596, 27.1261) -> (2.523, 27.6583) centre (-3.5862, 26.5485) ccw
  arc A340 (2.523, 27.6583) -> (2.3517, 28.4093) centre (-5.9205, 26.128) ccw
  arc A341 (2.3517, 28.4093) -> (2.0158, 29.431) centre (-8.3334, 25.4626) ccw
  arc A342 (0.4038, 27.247) -> (-0.4038, 27.247) centre (0, 0) ccw
  arc A343 (-2.596, 27.1261) -> (-3.3988, 27.0372) centre (0, 0) ccw
  arc A344 (-5.5644, 26.6758) -> (-6.3525, 26.4992) centre (0, 0) ccw
  arc A345 (-8.4651, 25.9018) -> (-9.229, 25.6396) centre (0, 0) ccw
  arc A346 (-11.2632, 24.8134) -> (-11.9936, 24.4687) centre (0, 0) ccw
  arc A347 (-13.9245, 23.4237) -> (-14.6125, 23.0008) centre (0, 0) ccw
  arc A348 (-16.4168, 21.7498) -> (-17.0541, 21.2537) centre (0, 0) ccw
  arc A349 (-18.7098, 19.8118) -> (-19.2887, 19.2486) centre (0, 0) ccw
  arc A350 (-20.7757, 17.6333) -> (-21.2891, 17.0099) centre (0, 0) ccw
  arc A351 (-22.5894, 15.2408) -> (-23.0312, 14.5646) centre (0, 0) ccw
  arc A352 (-24.1289, 12.6632) -> (-24.4936, 11.9426) centre (0, 0) ccw
  arc A353 (-25.3755, 9.932) -> (-25.6587, 9.1756) centre (0, 0) ccw
  arc A354 (-26.3141, 7.0802) -> (-26.5124, 6.2973) centre (0, 0) ccw
  arc A355 (-26.9333, 4.1425) -> (-27.0442, 3.3425) centre (0, 0) ccw
  arc A356 (-27.2255, 1.1544) -> (-27.2478, 0.3471) centre (0, 0) ccw
  arc A357 (-27.1873, -1.8476) -> (-27.1206, -2.6525) centre (0, 0) ccw
  arc A358 (-26.819, -4.8272) -> (-26.6642, -5.6199) centre (0, 0) ccw
  arc A359 (-26.1252, -7.7482) -> (-25.8841, -8.519) centre (0, 0) ccw
  arc A360 (-25.1143, -10.5752) -> (-24.7899, -11.3148) centre (0, 0) ccw
  arc A361 (-23.7985, -13.2738) -> (-23.3947, -13.9732) centre (0, 0) ccw
  arc A362 (-22.1938, -15.8113) -> (-21.7155, -16.462) centre (0, 0) ccw
  arc A363 (-20.3198, -18.1568) -> (-19.7728, -18.751) centre (0, 0) ccw
  arc A364 (-18.1991, -20.2819) -> (-17.59, -20.8124) centre (0, 0) ccw
  arc A365 (-15.8574, -22.1609) -> (-15.1937, -22.6211) centre (0, 0) ccw
  arc A366 (-13.3233, -23.7708) -> (-12.613, -24.1552) centre (0, 0) ccw
  arc A367 (-10.6274, -25.0922) -> (-9.8792, -25.3962) centre (0, 0) ccw
  arc A368 (-7.8026, -26.109) -> (-7.0254, -26.3288) centre (0, 0) ccw
  arc A369 (-4.883, -26.8089) -> (-4.0864, -26.9419) centre (0, 0) ccw
  arc A370 (-1.9042, -27.1834) -> (-1.0978, -27.2279) centre (0, 0) ccw
  arc A371 (1.0978, -27.2279) -> (1.9042, -27.1834) centre (0, 0) ccw
  arc A372 (4.0864, -26.9419) -> (4.883, -26.8089) centre (0, 0) ccw
  arc A373 (7.0254, -26.3288) -> (7.8026, -26.109) centre (0, 0) ccw
  arc A374 (9.8792, -25.3962) -> (10.6274, -25.0922) centre (0, 0) ccw
  arc A375 (12.613, -24.1552) -> (13.3233, -23.7708) centre (0, 0) ccw
  arc A376 (15.1937, -22.6211) -> (15.8574, -22.1609) centre (0, 0) ccw
  arc A377 (17.59, -20.8124) -> (18.1991, -20.2819) centre (0, 0) ccw
  arc A378 (19.7728, -18.751) -> (20.3198, -18.1568) centre (0, 0) ccw
  arc A379 (21.7155, -16.462) -> (22.1938, -15.8113) centre (0, 0) ccw
  arc A380 (23.3947, -13.9732) -> (23.7985, -13.2738) centre (0, 0) ccw
  arc A381 (24.7899, -11.3148) -> (25.1143, -10.5752) centre (0, 0) ccw
  arc A382 (25.8841, -8.519) -> (26.1252, -7.7482) centre (0, 0) ccw
  arc A383 (26.6642, -5.6199) -> (26.819, -4.8272) centre (0, 0) ccw
  arc A384 (27.1206, -2.6525) -> (27.1873, -1.8476) centre (0, 0) ccw
  arc A385 (27.2478, 0.3471) -> (27.2255, 1.1544) centre (0, 0) ccw
  arc A386 (27.0442, 3.3425) -> (26.9333, 4.1425) centre (0, 0) ccw
  arc A387 (26.5124, 6.2973) -> (26.3141, 7.0802) centre (0, 0) ccw
  arc A388 (25.6587, 9.1756) -> (25.3755, 9.932) centre (0, 0) ccw
  arc A389 (24.4936, 11.9426) -> (24.1289, 12.6632) centre (0, 0) ccw
  arc A390 (23.0312, 14.5646) -> (22.5894, 15.2408) centre (0, 0) ccw
  arc A391 (21.2891, 17.0099) -> (20.7757, 17.6333) centre (0, 0) ccw
  arc A392 (19.2887, 19.2486) -> (18.7098, 19.8118) centre (0, 0) ccw
  arc A393 (17.0541, 21.2537) -> (16.4168, 21.7498) centre (0, 0) ccw
  arc A394 (14.6125, 23.0008) -> (13.9245, 23.4237) centre (0, 0) ccw
  arc A395 (11.9936, 24.4687) -> (11.2632, 24.8134) centre (0, 0) ccw
  arc A396 (9.229, 25.6396) -> (8.4651, 25.9018) centre (0, 0) ccw
  arc A397 (6.3525, 26.4992) -> (5.5644, 26.6758) centre (0, 0) ccw
  arc A398 (3.3988, 27.0372) -> (2.596, 27.1261) centre (0, 0) ccw
  arc A399 (-1.2341, 29.4742) -> (-2.0158, 29.431) centre (0, 0) ccw
  arc A400 (-4.469, 29.1595) -> (-5.2412, 29.0307) centre (0, 0) ccw
  arc A401 (-7.6497, 28.4909) -> (-8.403, 28.2779) centre (0, 0) ccw
  arc A402 (-10.7375, 27.4765) -> (-11.4628, 27.1819) centre (0, 0) ccw
  arc A403 (-13.6949, 26.1285) -> (-14.3835, 25.7559) centre (0, 0) ccw
  arc A404 (-16.4862, 24.4634) -> (-17.1295, 24.0173) centre (0, 0) ccw
  arc A405 (-19.0773, 22.5013) -> (-19.6677, 21.9871) centre (0, 0) ccw
  arc A406 (-21.4368, 20.2661) -> (-21.9671, 19.69) centre (0, 0) ccw
  arc A407 (-23.5361, 17.7848) -> (-23.9998, 17.154) centre (0, 0) ccw
  arc A408 (-25.3498, 15.0877) -> (-25.7412, 14.4097) centre (0, 0) ccw
  arc A409 (-26.8557, 12.2075) -> (-27.1702, 11.4905) centre (0, 0) ccw
  arc A410 (-28.0356, 9.179) -> (-28.2693, 8.4318) centre (0, 0) ccw
  arc A411 (-28.8752, 6.0392) -> (-29.0253, 5.2708) centre (0, 0) ccw
  arc A412 (-29.3643, 2.826) -> (-29.429, 2.0458) centre (0, 0) ccw
  arc A413 (-29.497, -0.4215) -> (-29.4754, -1.2041) centre (0, 0) ccw
  arc A414 (-29.2716, -3.6638) -> (-29.1641, -4.4393) centre (0, 0) ccw
  arc A415 (-28.6909, -6.8617) -> (-28.4987, -7.6207) centre (0, 0) ccw
  arc A416 (-27.7619, -9.9763) -> (-27.4874, -10.7095) centre (0, 0) ccw
  arc A417 (-26.4959, -12.9698) -> (-26.1424, -13.6683) centre (0, 0) ccw
  arc A418 (-24.9083, -15.8058) -> (-24.4801, -16.4613) centre (0, 0) ccw
  arc A419 (-23.0184, -18.45) -> (-22.5207, -19.0544) centre (0, 0) ccw
  arc A420 (-20.849, -20.8703) -> (-20.2879, -21.4162) centre (0, 0) ccw
  arc A421 (-18.4266, -23.0372) -> (-17.8088, -23.518) centre (0, 0) ccw
  arc A422 (-15.7805, -24.9244) -> (-15.1135, -25.3344) centre (0, 0) ccw
  arc A423 (-12.9428, -26.5091) -> (-12.2348, -26.8433) centre (0, 0) ccw
  arc A424 (-9.948, -27.772) -> (-9.2075, -28.0263) centre (0, 0) ccw
  arc A425 (-6.8325, -28.6979) -> (-6.0685, -28.8691) centre (0, 0) ccw
  arc A426 (-3.634, -29.2753) -> (-2.8559, -29.3614) centre (0, 0) ccw
  arc A427 (-0.3915, -29.4974) -> (0.3915, -29.4974) centre (0, 0) ccw
  arc A428 (2.8559, -29.3614) -> (3.634, -29.2753) centre (0, 0) ccw
  arc A429 (6.0685, -28.8691) -> (6.8325, -28.6979) centre (0, 0) ccw
  arc A430 (9.2075, -28.0263) -> (9.948, -27.772) centre (0, 0) ccw
  arc A431 (12.2348, -26.8433) -> (12.9428, -26.5091) centre (0, 0) ccw
  arc A432 (15.1135, -25.3344) -> (15.7805, -24.9244) centre (0, 0) ccw
  arc A433 (17.8088, -23.518) -> (18.4266, -23.0372) centre (0, 0) ccw
  arc A434 (20.2879, -21.4162) -> (20.849, -20.8703) centre (0, 0) ccw
  arc A435 (22.5207, -19.0544) -> (23.0184, -18.45) centre (0, 0) ccw
  arc A436 (24.4801, -16.4613) -> (24.9083, -15.8058) centre (0, 0) ccw
  arc A437 (26.1424, -13.6683) -> (26.4959, -12.9698) centre (0, 0) ccw
  arc A438 (27.4874, -10.7095) -> (27.7619, -9.9763) centre (0, 0) ccw
  arc A439 (28.4987, -7.6207) -> (28.6909, -6.8617) centre (0, 0) ccw
  arc A440 (29.1641, -4.4393) -> (29.2716, -3.6638) centre (0, 0) ccw
  arc A441 (29.4754, -1.2041) -> (29.497, -0.4215) centre (0, 0) ccw
  arc A442 (29.429, 2.0458) -> (29.3643, 2.826) centre (0, 0) ccw
  arc A443 (29.0253, 5.2708) -> (28.8752, 6.0392) centre (0, 0) ccw
  arc A444 (28.2693, 8.4318) -> (28.0356, 9.179) centre (0, 0) ccw
  arc A445 (27.1702, 11.4905) -> (26.8557, 12.2075) centre (0, 0) ccw
  arc A446 (25.7412, 14.4097) -> (25.3498, 15.0877) centre (0, 0) ccw
  arc A447 (23.9998, 17.154) -> (23.5361, 17.7848) centre (0, 0) ccw
  arc A448 (21.9671, 19.69) -> (21.4368, 20.2661) centre (0, 0) ccw
  arc A449 (19.6677, 21.9871) -> (19.0773, 22.5013) centre (0, 0) ccw
  arc A450 (17.1295, 24.0173) -> (16.4862, 24.4634) centre (0, 0) ccw
  arc A451 (14.3835, 25.7559) -> (13.6949, 26.1285) centre (0, 0) ccw
  arc A452 (11.4628, 27.1819) -> (10.7375, 27.4765) centre (0, 0) ccw
  arc A453 (8.403, 28.2779) -> (7.6497, 28.4909) centre (0, 0) ccw
  arc A454 (5.2412, 29.0307) -> (4.469, 29.1595) centre (0, 0) ccw
  arc A455 (2.0158, 29.431) -> (1.2341, 29.4742) centre (0, 0) ccw
  line L0 (-31.5, 0) -> (31.5, 0)
  line L1 (0, -31.5) -> (0, 31.5)
  line L2 (49.5, 29.5) -> (119.5, 29.5)
  line L3 (49.5, 21.5) -> (119.5, 21.5)
  line L4 (49.5, 13.5) -> (119.5, 13.5)
  line L5 (49.5, 5.5) -> (119.5, 5.5)
  line L6 (49.5, -2.5) -> (119.5, -2.5)
  line L7 (49.5, -10.5) -> (119.5, -10.5)
  line L8 (49.5, -18.5) -> (119.5, -18.5)
  line L9 (49.5, -26.5) -> (119.5, -26.5)
  line L10 (49.5, -34.5) -> (119.5, -34.5)
  line L11 (49.5, -42.5) -> (119.5, -42.5)
  line L12 (49.5, -50.5) -> (119.5, -50.5)
  line L13 (49.5, -58.5) -> (119.5, -58.5)
  line L14 (49.5, -66.5) -> (119.5, -66.5)
  line L15 (49.5, 29.5) -> (49.5, -66.5)
  line L16 (119.5, 29.5) -> (119.5, -66.5)
  line L17 (84.5, 21.5) -> (84.5, -66.5)
  point P0 (0, 0)
  point P1 (55.5, 23.5)
  point P2 (58, 15.5)
  point P3 (58, 7.5)
  point P4 (55.5, -0.5)
  point P5 (58, -8.5)
  point P6 (53, -16.5)
  point P7 (55.5, -24.5)
  point P8 (55.5, -32.5)
  point P9 (55.5, -40.5)
  point P10 (58, -48.5)
  point P11 (58, -56.5)
  point P12 (55.5, -64.5)
  point P13 (85.5, 15.5)
  point P14 (100.5, 7.5)
  point P15 (101.75, -0.5)
  point P16 (98, -8.5)
  point P17 (100.5, -16.5)
  point P18 (94.25, -24.5)
  point P19 (100.5, -32.5)
  point P20 (98, -40.5)
  point P21 (95.5, -48.5)
  point P22 (1, 45)
  point P23 (1, 39)
  point P24 (17.1875, 45)
  point P25 (19.3125, 39)
  constraints: 684 point on circle, 342 centre point, 32 end point, 14 horizontal, 2 horizontal alignment, 2 midpoint, 2 vertical, 1591 other
extrude "押し出し2" add sketch "スケッチ2" along normal blind 4 contours A1 A2 A455 A341 A340 A339 A398 A168 A169 A170 A454 A338 A337 A336 A397 A165 A166 A167 A453 A335 A334 A333 A396 A162 A163 A164 A452 A332 A331 A330 A395 A159 A160 A161 A451 A329 A328 A327 A394 A156 A157 A158 A450 A326 A325 A324 A393 A153 A154 A155 A449 A323 A322 A321 A392 A150 A151 A152 A448 A320 A319 A318 A391 A147 A148 A149 A447 A317 A316 A315 A390 A144 A145 A146 A446 A314 A313 A312 A389 A141 A142 A143 A445 A311 A310 A309 A388 A138 A139 A140 A444 A308 A307 A306 A387 A135 A136 A137 A443 A305 A304 A303 A386 A132 A133 A134 A442 A302 A301 A300 A385 A129 A130 L0 L1 A342 A0 | L1 L0 A214 A213 A356 A42 A43 A44 A412 A212 A211 A210 A355 A39 A40 A41 A411 A209 A208 A207 A354 A36 A37 A38 A410 A206 A205 A204 A353 A33 A34 A35 A409 A203 A202 A201 A352 A30 A31 A32 A408 A200 A199 A198 A351 A27 A28 A29 A407 A197 A196 A195 A350 A24 A25 A26 A406 A194 A193 A192 A349 A21 A22 A23 A405 A191 A190 A189 A348 A18 A19 A20 A404 A188 A187 A186 A347 A15 A16 A17 A403 A185 A184 A183 A346 A12 A13 A14 A402 A182 A181 A180 A345 A9 A10 A11 A401 A179 A178 A177 A344 A6 A7 A8 A400 A176 A175 A174 A343 A3 A4 A5 A399 A173 A172 A171 A342 | L1 A427 A257 A256 A255 A370 A84 A85 A86 A426 A254 A253 A252 A369 A81 A82 A83 A425 A251 A250 A249 A368 A78 A79 A80 A424 A248 A247 A246 A367 A75 A76 A77 A423 A245 A244 A243 A366 A72 A73 A74 A422 A242 A241 A240 A365 A69 A70 A71 A421 A239 A238 A237 A364 A66 A67 A68 A420 A236 A235 A234 A363 A63 A64 A65 A419 A233 A232 A231 A362 A60 A61 A62 A418 A230 A229 A228 A361 A57 A58 A59 A417 A227 A226 A225 A360 A54 A55 A56 A416 A224 A223 A222 A359 A51 A52 A53 A415 A221 A220 A219 A358 A48 A49 A50 A414 A218 A217 A216 A357 A45 A46 A47 A413 A215 A214 L0 | L0 A130 A131 A441 A299 A298 A297 A384 A126 A127 A128 A440 A296 A295 A294 A383 A123 A124 A125 A439 A293 A292 A291 A382 A120 A121 A122 A438 A290 A289 A288 A381 A117 A118 A119 A437 A287 A286 A285 A380 A114 A115 A116 A436 A284 A283 A282 A379 A111 A112 A113 A435 A281 A280 A279 A378 A108 A109 A110 A434 A278 A277 A276 A377 A105 A106 A107 A433 A275 A274 A273 A376 A102 A103 A104 A432 A272 A271 A270 A375 A99 A100 A101 A431 A269 A268 A267 A374 A96 A97 A98 A430 A266 A265 A264 A373 A93 A94 A95 A429 A263 A262 A261 A372 A90 A91 A92 A428 A260 A259 A258 A371 A87 A88 A89 A427 L1
sketch "スケッチ3" plane through (0, 0, 8) normal (0, 0, 1) x (1, 0, 0)
  circle A0 centre (0, 0) radius 2.995
  dimension "d4" = 5.99
  constraints: 1 centre point, 1 coincident
  measures "d4" diameter of A0
extrude "押し出し3" cut sketch "スケッチ3" against normal through all